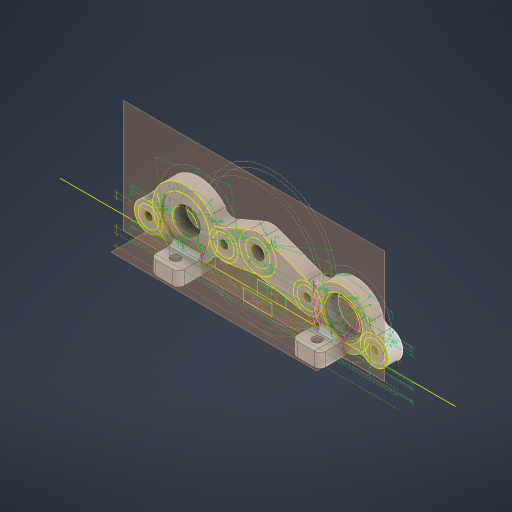
# Autodesk Inventor part: Motormount
Saved by Autodesk Inventor 2023.5 (Build 275446000, 446)
## iProperties
Created: 2024-12-07
Part Number: Motormount
Material: 一般
Document SubType Name: Modeling
Designer: IshiiLabHonda
Density: 1 g/cm^3
Appearance: 既定
Author: IshiiLabHonda
Autodesk Inventor part; units mm, degrees
ref_plane "YZ Plane" through (0, 0, 0) normal (1, 0, 0) x (0, 1, 0)
ref_plane "XZ Plane" through (0, 0, 0) normal (0, 1, 0) x (-1, 0, 0)
ref_plane "XY Plane" through (0, 0, 0) normal (0, 0, 1) x (1, 0, 0)
sketch "blueprint" plane through (0, 0, 0) normal (0, 0, 1) x (1, 0, 0)
  line L0 (0, 0) -> (0, 1) construction
  line L1 (0, 0) -> (1, 0) construction
  circle A0 centre (0, 0) radius 1.25
  circle A1 centre (0, 0) radius 11.5 construction
  line L2 (-25, -11.5) -> (25, -11.5) construction
  line L3 (-25, -9.5) -> (25, -9.5) construction
  line L4 (-25, -8.5) -> (25, -8.5) construction
  line L5 (-25, -4) -> (25, -4) construction
  circle A2 centre (0, 0) radius 10.65 construction
  circle A3 centre (-12.8817, -1.75) radius 2.25
  circle A4 centre (14.8916, -2.5) radius 4.35 construction
  circle A5 centre (14.8916, -2.5) radius 3.5 construction
  line L6 (-25, -3.2) -> (25, -3.2) construction
  circle A6 centre (-12.8817, -1.75) radius 4.25 construction
  circle A7 centre (-19.3421, -4.1014) radius 0.625 construction
  circle A8 centre (-6.0067, -1.75) radius 0.625 construction
  circle A9 centre (-12.8817, -1.75) radius 6.875 construction
  circle A10 centre (-19.3421, -4.1014) radius 1.825
  circle A11 centre (-6.0067, -1.75) radius 1.825
  circle A12 centre (14.8916, -2.5) radius 5
  circle A13 centre (14.8916, -2.5) radius 6.125 construction
  circle A14 centre (20.6472, -4.5949) radius 0.625 construction
  circle A15 centre (8.7666, -2.5) radius 0.625 construction
  circle A16 centre (20.6472, -4.5949) radius 1.825
  circle A17 centre (-19.3421, -4.1014) radius 0.8
  circle A18 centre (-6.0067, -1.75) radius 0.8
  circle A19 centre (20.6472, -4.5949) radius 0.8
  circle A20 centre (-19.3421, -4.1014) radius 2.5
  circle A21 centre (-6.0067, -1.75) radius 2.5
  circle A22 centre (20.6472, -4.5949) radius 2.5
  circle A23 centre (14.8916, -2.5) radius 3.6
  circle A24 centre (0, 0) radius 3.25
  line L7 (-15, -4) -> (-15, -8.5) construction
  line L8 (15, -4) -> (15, -8.5) construction
  line L9 (-10, -8.5) -> (-10, -6)
  line L10 (-15, -8.5) -> (-15, -6)
  line L11 (-15, -6) -> (-10, -6)
  line L12 (-12.5, -6) -> (-12.5, -8.5)
  line L13 (-13.3, -6) -> (-13.3, -8.5)
  line L14 (-11.7, -6) -> (-11.7, -8.5)
  line L15 (10, -8.5) -> (10, -6)
  line L16 (15, -8.5) -> (15, -6)
  line L17 (15, -6) -> (10, -6)
  line L18 (12.5, -6) -> (12.5, -8.5)
  line L19 (13.3, -6) -> (13.3, -8.5)
  line L20 (11.7, -6) -> (11.7, -8.5)
  line L21 (-15, -8.5) -> (-10, -8.5)
  line L22 (10, -8.5) -> (15, -8.5)
  circle A25 centre (8.7666, -2.5) radius 1.825
  line L23 (-12.8817, -1.75) -> (-19.3421, -4.1014) construction
  line L24 (-12.8817, -1.75) -> (-6.0067, -1.75) construction
  line L25 (14.8916, -2.5) -> (8.7666, -2.5) construction
  circle A26 centre (-12.8817, -1.75) radius 5.75
  line L26 (-2.5, -6.5) -> (2.5, -6.5)
  line L27 (2.5, -6.5) -> (2.5, -8.5)
  line L28 (2.5, -8.5) -> (-2.5, -8.5)
  line L29 (-2.5, -8.5) -> (-2.5, -6.5)
  line L30 (-2.5, -6.5) -> (2.5, -8.5) construction
  line L31 (2.5, -6.5) -> (-2.5, -8.5) construction
  line L32 (0, -6.5) -> (0, -8.5) construction
  line L33 (-0.8, -6.5) -> (-0.8, -8.5) construction
  line L34 (0.8, -6.5) -> (0.8, -8.5) construction
  circle A27 centre (8.7666, -2.5) radius 0.8
  circle A28 centre (8.7666, -2.5) radius 2.5
  line L35 (20.6472, -4.5949) -> (14.8916, -2.5) construction
  circle A29 centre (0, 0) radius 2.15
  circle A30 centre (14.8916, -2.5) radius 3 construction
  circle A31 centre (14.8916, -2.5) radius 3.2
  circle A32 centre (-12.8817, -1.75) radius 4.35
  point P0 (18.532, -5.9275)
  point P1 (19.8834, -2.2144)
  point P2 (0, -8.5)
  point P3 (-6.4807, -9.5)
  point P4 (6.4807, -9.5)
  point P5 (0, -7.5)
  point P6 (-17.257, -5.4808)
  point P7 (-7.4942, -3.7593)
  point P8 (-7.4942, 0.2593)
  point P9 (-18.6315, -1.7045)
  point P10 (11.284, 2.5721)
  point P11 (11.284, 2.0279)
  point P12 (16.9793, 5.3162)
  point P13 (16.5081, 5.5882)
  dimension "d0" = 1
  dimension "d1" = 1
  dimension "d2" = 2.5
  dimension "d3" = 23
  dimension "d4" = 50
  dimension "d5" = 50
  dimension "d6" = 2
  dimension "d7" = 50
  dimension "d9" = 1
  dimension "d10" = 50
  dimension "d12" = 4.5
  dimension "d13" = 21.3
  dimension "d14" = 4.5
  dimension "d15" = 8.7
  dimension "d17" = 0.1
  dimension "d18" = 0.1
  dimension "d20" = 7
  dimension "d21" = 50
  dimension "d22" = 0.8
  dimension "d23" = 8.5
  dimension "d26" = 1.25
  dimension "d27" = 1.25
  dimension "d28" = 1.2
  dimension "d29" = 1.2
  dimension "d31" = 1.5
  dimension "d32" = 1.25
  dimension "d33" = 1.25
  dimension "d34" = 1.2
  dimension "d37" = 0.5
  dimension "d40" = 1.6
  dimension "d41" = 1.6
  dimension "d43" = 1.6
  dimension "d49" = 2
  dimension "d56" = 30
  dimension "d90" = 2.5
  dimension "d92" = 5
  dimension "d93" = 1.6
  dimension "d104" = 1.2
  dimension "d105" = 5
  dimension "d106" = 1.6
  dimension "d107" = 2.5
  dimension "d129" = 5
  dimension "d130" = 5
  dimension "d132" = 5
  dimension "d155" = 25
  dimension "d158" = 1.5
  dimension "d160" = 0.5
  dimension "d161" = 200
  dimension "d166" = 1.6
  dimension "d167" = 5
  dimension "d168" = 2
  dimension "d178" = 1.6
  dimension "d179" = 5
  dimension "d187" = -2.8
  dimension "d196" = 4.3
  dimension "d218" = 12.0639
  dimension "d219" = 13.5411
  dimension "d220" = 200
  dimension "d237" = 0.1
  dimension "d238" = 6
  dimension "d239" = 0.2
  dimension "d247" = 0.1
  dimension "d257" = 9.75
  dimension "d258" = 9
  constraints: 70 end point, 33 centre point, 28 coincident, 16 point on line, 10 parallel, 8 midpoint, 7 vertical, 6 point on circle, 5 symmetric about line, 4 perpendicular, 3 horizontal, 1 tangent, 18 other
  measures "d0" distance of L0.start L0.end
  measures "d1" distance of L0.start L1.end
  measures "d2" diameter of A0
  measures "d3" diameter of A1
  measures "d4" distance of L2.start L2.end
  measures "d5" distance of L3.start L3.end
  measures "d6" distance between parallel lines of L2 L3
  measures "d7" distance of point (-25, -8.5) point (25, -8.5)
  measures "d10" distance of L5.start L5.end
  measures "d13" diameter of A2
  measures "d14" diameter of A3
  measures "d15" diameter of A4
  measures "d20" diameter of A5
  measures "d21" distance of L6.start L6.end
  measures "d22" distance between parallel lines of L5 L6
  measures "d23" diameter of A6
  measures "d26" diameter of A8
  measures "d27" diameter of A7
  measures "d28" radial gap between concentric circles of A10 A7
  measures "d29" radial gap between concentric circles of A11 A8
  measures "d31" radial gap between concentric circles of A12 A5
  measures "d32" diameter of A14
  measures "d33" diameter of A15
  measures "d34" radial gap between concentric circles of A14 A16
  measures "d40" diameter of A17
  measures "d41" diameter of A18
  measures "d43" diameter of A19
  measures "d49" radial gap between concentric circles of A24 A0
  measures "d56" distance between parallel lines of L8 L7
  measures "d90" distance of L10.start L10.end
  measures "d92" distance between parallel lines of L9 L10
  measures "d93" distance between parallel lines of L14 L13
  measures "d104" radial gap between concentric circles of A25 A15
  measures "d105" distance between parallel lines of L16 L15
  measures "d106" distance between parallel lines of L19 L20
  measures "d107" distance of L15.start L15.end
  measures "d129" diameter of A20
  measures "d130" diameter of A21
  measures "d132" diameter of A22
  measures "d155" distance between parallel lines of L18 L12
  measures "d158" radial gap between concentric circles of A26 A6
  measures "d166" distance between parallel lines of L33 L34
  measures "d167" distance between parallel lines of L27 L29
  measures "d168" distance between parallel lines of L26 L28
  measures "d178" diameter of A27
  measures "d179" diameter of A28
  measures "d187" distance edge to line of A6 L6
  measures "d196" diameter of A29
  measures "d218" distance of A14.centre L25.end
  measures "d219" distance of A7.centre A18.centre
  measures "d237" radial gap between concentric circles of A5 A23
  measures "d238" diameter of A30
  measures "d239" radial gap between concentric circles of A30 A31
  measures "d247" radial gap between concentric circles of A6 A32
  measures "d257" distance from line of L2 A3.centre
  measures "d258" distance from line of L2 A4.centre
sketch "スケッチ5" plane through (0, 0, 0) normal (0, 0, 1) x (1, 0, 0)
  circle A0 centre (0, 0) radius 10.65 construction
  circle A1 centre (0, 0) radius 11.5 construction
  line L0 (-25, -3.2) -> (25, -3.2) construction
  line L1 (-25, -4) -> (25, -4) construction
  line L2 (-25, -8.5) -> (25, -8.5) construction
  line L3 (-25, -9.5) -> (25, -9.5) construction
  line L4 (-25, -11.5) -> (25, -11.5) construction
  line L5 (0, 0) -> (1, 0) construction
  circle A2 centre (0, 0) radius 1.25 projected
  line L6 (0, 0) -> (0, 1) construction
  circle A3 centre (-6.0067, -1.75) radius 0.625 construction
  circle A4 centre (-6.0067, -1.75) radius 0.8 projected
  circle A5 centre (-6.0067, -1.75) radius 1.825 construction
  circle A6 centre (-6.0067, -1.75) radius 2.5 projected
  line L7 (-12.8817, -1.75) -> (-6.0067, -1.75) construction
  circle A7 centre (-12.8817, -1.75) radius 2.25 projected
  circle A8 centre (-12.8817, -1.75) radius 4.25 construction
  circle A9 centre (-12.8817, -1.75) radius 5.75 projected
  circle A10 centre (-12.8817, -1.75) radius 6.875 construction
  line L8 (-12.8817, -1.75) -> (-19.3421, -4.1014) construction
  circle A11 centre (-19.3421, -4.1014) radius 2.5 projected
  circle A12 centre (14.8916, -2.5) radius 3.5 construction
  circle A13 centre (14.8916, -2.5) radius 4.35 construction
  circle A14 centre (-19.3421, -4.1014) radius 0.625 construction
  circle A15 centre (-19.3421, -4.1014) radius 0.8 projected
  circle A16 centre (-19.3421, -4.1014) radius 1.825 construction
  circle A17 centre (14.8916, -2.5) radius 5 projected
  circle A18 centre (14.8916, -2.5) radius 6.125 construction
  circle A19 centre (20.6472, -4.5949) radius 0.625 construction
  circle A20 centre (8.7666, -2.5) radius 0.625 construction
  circle A21 centre (20.6472, -4.5949) radius 1.825 construction
  line L9 (14.8916, -2.5) -> (8.7666, -2.5) construction
  circle A22 centre (8.7666, -2.5) radius 0.8 projected
  circle A23 centre (8.7666, -2.5) radius 1.825 construction
  circle A24 centre (8.7666, -2.5) radius 2.5 projected
  circle A25 centre (14.8916, -2.5) radius 3.6 projected
  line L10 (20.6472, -4.5949) -> (14.8916, -2.5) construction
  circle A26 centre (20.6472, -4.5949) radius 2.5 projected
  circle A27 centre (20.6472, -4.5949) radius 0.8 projected
  line L11 (-10, -8.5) -> (-10, -6) projected
  line L12 (-11.7, -6) -> (-11.7, -8.5) projected
  line L13 (-15, -6) -> (-10, -6) projected
  line L14 (-12.5, -6) -> (-12.5, -8.5) projected
  line L15 (-13.3, -6) -> (-13.3, -8.5) projected
  line L16 (-15, -8.5) -> (-10, -8.5) projected
  line L17 (-15, -4) -> (-15, -8.5) construction
  line L18 (-15, -8.5) -> (-15, -6) projected
  line L19 (15, -4) -> (15, -8.5) construction
  line L20 (15, -8.5) -> (15, -6) projected
  line L21 (13.3, -6) -> (13.3, -8.5) projected
  line L22 (15, -6) -> (10, -6) projected
  line L23 (12.5, -6) -> (12.5, -8.5) projected
  line L24 (11.7, -6) -> (11.7, -8.5) projected
  line L25 (10, -8.5) -> (15, -8.5) projected
  line L26 (10, -8.5) -> (10, -6) projected
  circle A28 centre (0, 0) radius 3.25 projected
  line L27 (-2.5, -8.5) -> (-2.5, -6.5) projected
  line L28 (-0.8, -6.5) -> (-0.8, -8.5) construction
  line L29 (0, -6.5) -> (0, -8.5) construction
  line L30 (0.8, -6.5) -> (0.8, -8.5) construction
  line L31 (-2.5, -6.5) -> (2.5, -6.5) projected
  line L32 (-2.5, -6.5) -> (2.5, -8.5) construction
  line L33 (2.5, -6.5) -> (-2.5, -8.5) construction
  line L34 (2.5, -8.5) -> (-2.5, -8.5) projected
  line L35 (2.5, -6.5) -> (2.5, -8.5) projected
  line L36 (-15, -6) -> (-17.9261, 0.4132)
  line L37 (-10, -6) -> (-7.3501, 0.6797)
  line L38 (10, -6) -> (9.8941, -2.6584)
  line L39 (15, -6) -> (19.0045, 0.0357)
  line L40 (-5.6002, -4.2167) -> (0.5285, -3.2067)
  line L41 (-6.9886, 0.5491) -> (-1.2766, 2.9888)
  line L42 (1.1454, 3.0415) -> (9.6477, -0.1604)
  line L43 (-0.6311, -3.1881) -> (8.2811, -4.9524)
  point P0 (0, -7.5)
  point P1 (0, -8.5)
  point P2 (6.4807, -9.5)
  point P3 (-6.4807, -9.5)
  point P4 (10.2985, -4.4757)
  point P5 (9.9587, -4.6975)
  point P6 (0.8824, 3.1335)
  point P7 (-18.6315, -1.7045)
  point P8 (-17.257, -5.4808)
  point P9 (-7.4942, -3.7593)
  point P10 (18.532, -5.9275)
  point P11 (19.8834, -2.2144)
  point P12 (10.2985, -0.5243)
  point P13 (-7.4942, 0.2593)
  point P14 (18.0158, -1.9266)
  point P15 (-17.2201, -1.1342)
  point P16 (15, -7.4988)
  point P17 (11.3209, -6)
  point P18 (-0.053, -3.3026)
  point P19 (-15, -7.0956)
  point P20 (-10, -6.7258)
  point P21 (-7.5052, 0.2887)
  constraints: 16 end point, 8 point on circle, 8 tangent, 15 other
extrude "押し出し33" add sketch "スケッチ5" along normal blind 2.5 contours A6 A9 | A6 L41 A28 L43 L40 | A9 A6 L37 | A6 L37 A9 | A28 | A9 L11 L37 A6 | L40 A28 L42 A24 L43 | L37 A6 | A6 L37 L13 L18 A9 A11 | A9 L12 L13 L11 | A24 A17 L38 | A11 A9 | A9 A11 | A9 L14 L13 L12 | L38 A17 A24 | A24 A17 | A17 A26 L20 A25 L22 A24 | A9 L15 L13 L14 | L18 L13 L15 A9 | A26 A17 | A17 A26 | L22 L24 A17 | L24 L22 L23 A17 | A17 L21 L22 A25 L20 | L23 L22 L21 A17 | L20 L39 A25 | A25 L22 L20 | A25 L39 L22 | A7 | A15 | A27
extrude "押し出し34" cut sketch "blueprint" along normal blind 0.5 contours A10 A26 | A26 A10 | A26 A11 | A11 A26 | A16 A12 | A12 A16 | A25 A12 | A12 A25 | A17 | A19 | A29
extrude "押し出し39" add sketch "blueprint" along normal blind 6.5 contours A26 L13 L21 L10 | L10 L11 A32 L13 A26 | A26 L12 L21 L13 | L13 A32 L12 A26 | A26 L14 L11 L9 | L9 L21 L14 A26 | L11 L13 A32 | L13 L11 L12 A32 | A26 L14 L21 L12 | L12 A32 L11 L14 A26 | L12 L11 A32 | L16 L22 L19 A12 | A12 L19 L17 A23 L16 | L17 L20 A12 | A12 L20 L22 L15 L17 | L19 L22 L18 A12 | A12 L18 L17 L19 | A23 L17 L16 | L20 L17 L18 A12 | A12 L18 L22 L20 picked at (14.4705, -6.0203)
ref_plane "作業平面8" through (-15, -6, 2.5) normal (0, 1, 0) x (1, 0, 0)
sketch "スケッチ9" plane through (-15, -6, 2.5) normal (0, 1, 0) x (1, 0, 0)
  line L0 (0, 0) -> (5, 0) projected
  line L1 (0, 0) -> (0, -4) projected
  line L2 (5, -4) -> (0, -4) projected
  line L3 (5, 0) -> (5, -4) projected
  line L4 (26.3209, 0) -> (30, 0) projected
  line L5 (25, 2.5) -> (25, -4) projected
  line L6 (30, -4) -> (25, -4) projected
  line L7 (30, 0) -> (30, -4) projected
  line L8 (0, 2.5) -> (0, 0) projected
  line L9 (5, 2.5) -> (5, -4) projected
  line L10 (0, 0) -> (5, -4) construction
  line L11 (0, 2.5) -> (0, -4) projected
  line L12 (5, 0) -> (5.3524, 0) projected
  line L13 (0, -4) -> (5, 0) construction
  line L14 (30, 2.5) -> (30, -4) projected
  line L15 (25, 0) -> (30, -4) construction
  line L16 (25, 2.5) -> (25, -4) projected
  line L17 (30, 0) -> (30, 2.5) projected
  line L18 (25, -4) -> (30, 0) construction
  circle A0 centre (2.5, -2) radius 0.8
  circle A1 centre (27.5, -2) radius 0.8
  line L19 (26.3209, 2.5) -> (26.3209, 0) projected
  line L20 (26.3209, 2.5) -> (25, 2.5) projected
  point P0 (15, 2.5)
  dimension "d227" = 1.6
  dimension "d228" = 1.6
  constraints: 8 end point, 2 centre point, 2 midpoint
  measures "d227" diameter of A0
  measures "d228" diameter of A1
extrude "押し出し40" cut sketch "スケッチ9" against normal blind 6.5 contours A0 | A1
fillet "フィレット8" radius 1 4 edges at (-15, -7.25, 6.5) (-10, -7.25, 6.5) (10, -7.25, 6.5) (15, -7.25, 6.5)
fillet "フィレット9" radius 0.8 2 edges at (-12.5, -6, 2.5) (13.1604, -6, 2.5)
extrude "押し出し41" cut sketch "スケッチ5" along normal blind 6.5 contours A27
extrude "押し出し42" cut sketch "blueprint" along normal blind 6.5 contours L16 L17 A23 | A23 L17 L16 | A31
extrude "押し出し43" add sketch "blueprint" along normal up to surface (2.5 mm away) contours L16 L17 A23 | A23 L17 L16
ref_plane "作業平面9" through (0, 0, 2.5) normal (0, 0, 1) x (1, 0, 0)
sketch "スケッチ10" plane through (0, 0, 2.5) normal (0, 0, 1) x (1, 0, 0)
  line L0 (-1.2766, 2.9888) -> (-6.9886, 0.5491) projected
  arc A0 (-6.9886, 0.5491) -> (-7.4942, 0.2593) centre (-6.0067, -1.75) ccw projected
  line L1 (-1.2766, 2.9888) -> (-6.9886, 0.5491) projected
  line L2 (-5.6002, -4.2167) -> (0.5285, -3.2067) projected
  line L3 (-5.6002, -4.2167) -> (0.5285, -3.2067) projected
  circle A1 centre (-6.0067, -1.75) radius 0.8 projected
  circle A2 centre (-6.0067, -1.75) radius 0.8 projected
  circle A3 centre (-6.0067, -1.75) radius 1.825 projected
  circle A4 centre (-6.0067, -1.75) radius 1.825 projected
  arc A5 (-6.9886, 0.5491) -> (-7.4942, 0.2593) centre (-6.0067, -1.75) ccw projected
  arc A6 (-7.4942, -3.7593) -> (-5.6002, -4.2167) centre (-6.0067, -1.75) ccw projected
  arc A7 (-17.257, -5.4808) -> (-15, -7.0956) centre (-12.8817, -1.75) ccw projected
  arc A8 (-7.4942, -3.7593) -> (-5.6002, -4.2167) centre (-6.0067, -1.75) ccw projected
  arc A9 (-17.257, -5.4808) -> (-15, -7.0956) centre (-12.8817, -1.75) ccw projected
  arc A10 (0.5285, -3.2067) -> (-0.6311, -3.1881) centre (0, 0) ccw projected
  circle A11 centre (0, 0) radius 1.25 projected
  circle A12 centre (0, 0) radius 1.25 projected
  circle A13 centre (0, 0) radius 2.15 projected
  circle A14 centre (0, 0) radius 2.15 projected
  arc A15 (0.5285, -3.2067) -> (-0.6311, -3.1881) centre (0, 0) ccw projected
  arc A16 (0.5285, -3.2067) -> (-0.6311, -3.1881) centre (0, 0) ccw projected
  arc A17 (0.5285, -3.2067) -> (-0.6311, -3.1881) centre (0, 0) ccw projected
  line L4 (-0.6311, -3.1881) -> (8.2811, -4.9524) projected
  line L5 (9.6477, -0.1604) -> (1.1454, 3.0415) projected
  line L6 (9.6477, -0.1604) -> (1.1454, 3.0415) projected
  circle A18 centre (8.7666, -2.5) radius 0.8 projected
  circle A19 centre (8.7666, -2.5) radius 0.8 projected
  line L7 (-0.6311, -3.1881) -> (8.2811, -4.9524) projected
  line L8 (-15, -8.5) -> (-10, -8.5) projected
  line L9 (-10, -8.5) -> (-10, -6.9556) projected
  line L10 (-10, -6) -> (-10, -5.2) projected
  arc A20 (-15, -7.0868) -> (-15.4511, -5.0113) centre (-20, -7.0868) ccw projected
  arc A21 (-15, -7.0868) -> (-15.4511, -5.0113) centre (-20, -7.0868) ccw projected
  line L11 (-15, -7.0956) -> (-15, -5.2) projected
  line L12 (-10, -8.5) -> (-10, -6) projected
  line L13 (-15, -5.2) -> (-15, -6) projected
  line L14 (-15, -6) -> (-10, -6) projected
  line L15 (-11, -6) -> (-11, -8.5) projected
  line L16 (-10, -8.5) -> (-11, -8.5) projected
  line L17 (-11, -6) -> (-14, -6) projected
  line L18 (-14, -8.5) -> (-11, -8.5) projected
  line L19 (-15, -6) -> (-15, -8.5) projected
  line L20 (-14, -8.5) -> (-14, -6) projected
  line L21 (-15, -6) -> (-14, -6) projected
  line L22 (-15, -7.0868) -> (-15, -8.5) projected
  arc A22 (10.2985, -0.5243) -> (9.6477, -0.1604) centre (8.7666, -2.5) ccw projected
  arc A23 (19.8834, -2.2144) -> (10.2985, -0.5243) centre (14.8916, -2.5) ccw projected
  arc A24 (18.532, -5.9275) -> (19.8834, -2.2144) centre (20.6472, -4.5949) ccw projected
  arc A25 (19.8834, -2.2144) -> (10.2985, -0.5243) centre (14.8916, -2.5) ccw projected
  arc A26 (10.2985, -0.5243) -> (9.6477, -0.1604) centre (8.7666, -2.5) ccw projected
  circle A27 centre (20.6472, -4.5949) radius 1.825 projected
  circle A28 centre (20.6472, -4.5949) radius 1.825 projected
  circle A29 centre (14.8916, -2.5) radius 3.2 projected
  circle A30 centre (14.8916, -2.5) radius 3.2 projected
  arc A31 (10.2985, -4.4757) -> (10.6833, -5.2) centre (14.8916, -2.5) ccw projected
  arc A32 (10.2985, -0.5243) -> (9.6477, -0.1604) centre (8.7666, -2.5) ccw projected
  arc A33 (19.8834, -2.2144) -> (10.2985, -0.5243) centre (14.8916, -2.5) ccw projected
  circle A34 centre (20.6472, -4.5949) radius 0.8 projected
  arc A35 (18.532, -5.9275) -> (19.8834, -2.2144) centre (20.6472, -4.5949) ccw projected
  circle A36 centre (20.6472, -4.5949) radius 0.8 projected
  line L23 (-10, -5.2) -> (-10, -6.7258) projected
  arc A37 (-9.6476, -5.1118) -> (-10, -6.9556) centre (-5, -6.9556) ccw projected
  arc A38 (-9.6476, -5.1118) -> (-10, -6.9556) centre (-5, -6.9556) ccw projected
  line L24 (-14, -8.5) -> (-15, -8.5) projected
  line L25 (-11.7, -8.5) -> (-13.3, -8.5) projected
  line L26 (-13.3, -6) -> (-11.7, -6) projected
  line L27 (9.8782, 0.5881) -> (10.0005, -6.0244) projected
  line L28 (10, -8.5) -> (15, -8.5) projected
  line L29 (15, -8.5) -> (15, -7.5078) projected
  line L30 (15.8336, -4.7436) -> (19.0045, 0.0357) projected
  arc A39 (15.8336, -4.7436) -> (15, -7.5078) centre (20, -7.5078) ccw projected
  line L31 (15.8336, -4.7436) -> (19.0045, 0.0357) projected
  arc A40 (8.2811, -4.9524) -> (10.2985, -4.4757) centre (8.7666, -2.5) ccw projected
  line L32 (15, -6) -> (15, -5.2) projected
  line L33 (9.8782, 0.5881) -> (9.9852, -5.2) projected
  arc A41 (15.8336, -4.7436) -> (15, -7.5078) centre (20, -7.5078) ccw projected
  line L34 (15, -5.2) -> (15, -7.5078) projected
  line L35 (12.5104, -5.2) -> (10.6833, -5.2) projected
  line L36 (11.7, -6) -> (13.3, -6) projected
  line L37 (11.3209, -6) -> (14.049, -6) projected
  line L38 (9.9852, -5.2) -> (10.0005, -6.0244) projected
  line L39 (15, -8.5) -> (15, -6) projected
  line L40 (13.3, -8.5) -> (11.7, -8.5) projected
  line L41 (10, -6) -> (10, -8.5) projected
  line L42 (10, -6) -> (10, -8.5) projected
  arc A42 (-7.4942, 0.2593) -> (-18.6315, -1.7045) centre (-12.8817, -1.75) ccw projected
  arc A43 (-18.6315, -1.7045) -> (-17.257, -5.4808) centre (-19.3421, -4.1014) ccw projected
  line L43 (-17.9261, 0.4132) -> (-15.4511, -5.0113) projected
  circle A44 centre (-19.3421, -4.1014) radius 1.825 projected
  circle A45 centre (-19.3421, -4.1014) radius 1.825 projected
  circle A46 centre (8.7666, -2.5) radius 1.825 projected
  circle A47 centre (8.7666, -2.5) radius 1.825 projected
  line L44 (-9.6476, -5.1118) -> (-7.3501, 0.6797) projected
  line L45 (-9.6476, -5.1118) -> (-7.3501, 0.6797) projected
  arc A48 (-7.4942, 0.2593) -> (-18.6315, -1.7045) centre (-12.8817, -1.75) ccw projected
  line L46 (-17.9261, 0.4132) -> (-15.4511, -5.0113) projected
  arc A49 (-18.6315, -1.7045) -> (-17.257, -5.4808) centre (-19.3421, -4.1014) ccw projected
  line L47 (-10, -5.2) -> (-15, -5.2) projected
  line L48 (-11, -6) -> (-10, -6) projected
  line L49 (11, -8.5) -> (10, -8.5) projected
  line L50 (11, -8.5) -> (14, -8.5) projected
  line L51 (11, -8.5) -> (11, -6) projected
  line L52 (15, -8.5) -> (14, -8.5) projected
  line L53 (14, -6) -> (14, -8.5) projected
  line L54 (14, -6) -> (15, -6) projected
  line L55 (14, -6) -> (11, -6) projected
  line L56 (11.3209, -6) -> (11, -6) projected
  line L57 (-35, -6) -> (35, -6) projected
  line L58 (-25, -3.2) -> (25, -3.2) construction
  line L59 (-25, -4) -> (25, -4) construction
  line L60 (-25, -8.5) -> (25, -8.5) construction
  line L61 (-25, -9.5) -> (25, -9.5) construction
  line L62 (-25, -11.5) -> (25, -11.5) construction
  circle A50 centre (0, 0) radius 10.65 construction
  circle A51 centre (0, 0) radius 11.5 construction
  circle A52 centre (0, 0) radius 1.25 projected
  circle A53 centre (0, 0) radius 3.25 projected
  line L63 (-2.5, -8.5) -> (-2.5, -6.5) projected
  line L64 (-0.8, -6.5) -> (-0.8, -8.5) construction
  circle A54 centre (0, 0) radius 2.15 projected
  line L65 (0, -6.5) -> (0, -8.5) construction
  line L66 (0.8, -6.5) -> (0.8, -8.5) construction
  line L67 (-2.5, -6.5) -> (2.5, -6.5) projected
  line L68 (2.5, -8.5) -> (-2.5, -8.5) projected
  line L69 (2.5, -6.5) -> (-2.5, -8.5) construction
  line L70 (-2.5, -6.5) -> (2.5, -8.5) construction
  circle A55 centre (-6.0067, -1.75) radius 0.625 construction
  circle A56 centre (-6.0067, -1.75) radius 0.8 projected
  circle A57 centre (-6.0067, -1.75) radius 1.825 projected
  circle A58 centre (-6.0067, -1.75) radius 2.5 projected
  line L71 (-15, -4) -> (-15, -8.5) construction
  line L72 (-15, -8.5) -> (-15, -6) projected
  line L73 (-13.3, -6) -> (-13.3, -8.5) projected
  line L74 (-12.5, -6) -> (-12.5, -8.5) projected
  line L75 (-15, -6) -> (-10, -6) projected
  line L76 (-11.7, -6) -> (-11.7, -8.5) projected
  line L77 (-15, -8.5) -> (-10, -8.5) projected
  line L78 (-10, -8.5) -> (-10, -6) projected
  circle A59 centre (-12.8817, -1.75) radius 2.25 projected
  circle A60 centre (-12.8817, -1.75) radius 4.25 construction
  line L79 (-12.8817, -1.75) -> (-6.0067, -1.75) construction
  circle A61 centre (-12.8817, -1.75) radius 5.75 projected
  line L80 (-12.8817, -1.75) -> (-19.3421, -4.1014) construction
  circle A62 centre (-19.3421, -4.1014) radius 0.625 construction
  circle A63 centre (-19.3421, -4.1014) radius 1.825 projected
  circle A64 centre (-19.3421, -4.1014) radius 2.5 projected
  circle A65 centre (-19.3421, -4.1014) radius 0.8 projected
  line L81 (2.5, -6.5) -> (2.5, -8.5) projected
  line L82 (15, -6) -> (10, -6) projected
  line L83 (10, -8.5) -> (10, -6) projected
  line L84 (10, -8.5) -> (15, -8.5) projected
  line L85 (15, -4) -> (15, -8.5) construction
  line L86 (15, -8.5) -> (15, -6) projected
  line L87 (11.7, -6) -> (11.7, -8.5) projected
  line L88 (12.5, -6) -> (12.5, -8.5) projected
  line L89 (13.3, -6) -> (13.3, -8.5) projected
  circle A66 centre (14.8916, -2.5) radius 5 projected
  circle A67 centre (14.8916, -2.5) radius 6.125 construction
  circle A68 centre (20.6472, -4.5949) radius 0.625 construction
  circle A69 centre (8.7666, -2.5) radius 0.625 construction
  circle A70 centre (20.6472, -4.5949) radius 1.825 projected
  circle A71 centre (20.6472, -4.5949) radius 0.8 projected
  circle A72 centre (20.6472, -4.5949) radius 2.5 projected
  line L90 (14.8916, -2.5) -> (8.7666, -2.5) construction
  circle A73 centre (8.7666, -2.5) radius 1.825 projected
  circle A74 centre (8.7666, -2.5) radius 2.5 projected
  circle A75 centre (14.8916, -2.5) radius 3 construction
  circle A76 centre (14.8916, -2.5) radius 3.2 projected
  circle A77 centre (14.8916, -2.5) radius 3.6 projected
  line L91 (20.6472, -4.5949) -> (14.8916, -2.5) construction
  circle A78 centre (8.7666, -2.5) radius 0.8 projected
  line L92 (0, 0) -> (0, 1) construction
  line L93 (0, 0) -> (1, 0) construction
  circle A79 centre (14.8916, -2.5) radius 3.5 construction
  circle A80 centre (14.8916, -2.5) radius 4.35 construction
  line L94 (12.5, -6) -> (12.5, -8.5) projected
  line L95 (11.7, -6) -> (11.7, -8.5) projected
  line L96 (13.3, -6) -> (13.3, -8.5) projected
  line L97 (10, -8.5) -> (10, -6) projected
  line L98 (10, -8.5) -> (15, -8.5) projected
  line L99 (15, -4) -> (15, -8.5) construction
  line L100 (15, -6) -> (10, -6) projected
  line L101 (15, -6) -> (19.0045, 0.0357) projected
  line L102 (10, -6) -> (9.8941, -2.6584) projected
  line L103 (14.8916, -2.5) -> (8.7666, -2.5) construction
  line L104 (-0.6311, -3.1881) -> (8.2811, -4.9524) projected
  line L105 (1.1454, 3.0415) -> (9.6477, -0.1604) projected
  circle A81 centre (0, 0) radius 10.65 construction
  circle A82 centre (0, 0) radius 11.5 construction
  line L106 (-25, -11.5) -> (25, -11.5) construction
  line L107 (-25, -9.5) -> (25, -9.5) construction
  line L108 (-25, -8.5) -> (25, -8.5) construction
  line L109 (-25, -4) -> (25, -4) construction
  line L110 (-25, -3.2) -> (25, -3.2) construction
  circle A83 centre (8.7666, -2.5) radius 0.625 construction
  circle A84 centre (8.7666, -2.5) radius 0.8 projected
  circle A85 centre (8.7666, -2.5) radius 1.825 construction
  circle A86 centre (8.7666, -2.5) radius 2.5 projected
  line L111 (-15, -6) -> (-17.9261, 0.4132) projected
  line L112 (-10, -6) -> (-7.3501, 0.6797) projected
  line L113 (-12.8817, -1.75) -> (-6.0067, -1.75) construction
  circle A87 centre (-19.3421, -4.1014) radius 0.625 construction
  circle A88 centre (-19.3421, -4.1014) radius 0.8 projected
  circle A89 centre (-19.3421, -4.1014) radius 1.825 construction
  circle A90 centre (-19.3421, -4.1014) radius 2.5 projected
  line L114 (-12.8817, -1.75) -> (-19.3421, -4.1014) construction
  circle A91 centre (-12.8817, -1.75) radius 5.75 projected
  circle A92 centre (-12.8817, -1.75) radius 4.25 construction
  circle A93 centre (-12.8817, -1.75) radius 2.25 projected
  circle A94 centre (14.8916, -2.5) radius 3.5 construction
  circle A95 centre (14.8916, -2.5) radius 4.35 construction
  circle A96 centre (14.8916, -2.5) radius 5 projected
  circle A97 centre (14.8916, -2.5) radius 6.125 construction
  circle A98 centre (20.6472, -4.5949) radius 0.625 construction
  circle A99 centre (20.6472, -4.5949) radius 1.825 construction
  circle A100 centre (14.8916, -2.5) radius 3.6 projected
  line L115 (20.6472, -4.5949) -> (14.8916, -2.5) construction
  circle A101 centre (20.6472, -4.5949) radius 0.8 projected
  circle A102 centre (20.6472, -4.5949) radius 2.5 projected
  line L116 (-15, -6) -> (-10, -6) projected
  line L117 (-15, -4) -> (-15, -8.5) construction
  line L118 (-15, -8.5) -> (-10, -8.5) projected
  line L119 (-15, -8.5) -> (-15, -6) projected
  line L120 (-13.3, -6) -> (-13.3, -8.5) projected
  line L121 (-12.5, -6) -> (-12.5, -8.5) projected
  line L122 (-11.7, -6) -> (-11.7, -8.5) projected
  line L123 (-10, -8.5) -> (-10, -6) projected
  line L124 (0, 0) -> (1, 0) construction
  circle A103 centre (0, 0) radius 1.25 projected
  line L125 (0, 0) -> (0, 1) construction
  circle A104 centre (-6.0067, -1.75) radius 0.625 construction
  circle A105 centre (-6.0067, -1.75) radius 0.8 projected
  circle A106 centre (-6.0067, -1.75) radius 1.825 construction
  circle A107 centre (-6.0067, -1.75) radius 2.5 projected
  line L126 (-5.6002, -4.2167) -> (0.5285, -3.2067) projected
  line L127 (-2.5, -8.5) -> (-2.5, -6.5) projected
  line L128 (-0.8, -6.5) -> (-0.8, -8.5) construction
  line L129 (0, -6.5) -> (0, -8.5) construction
  line L130 (0.8, -6.5) -> (0.8, -8.5) construction
  line L131 (-6.9886, 0.5491) -> (-1.2766, 2.9888) projected
  circle A108 centre (0, 0) radius 3.25 projected
  line L132 (2.5, -6.5) -> (2.5, -8.5) projected
  line L133 (-2.5, -6.5) -> (2.5, -8.5) construction
  line L134 (2.5, -6.5) -> (-2.5, -8.5) construction
  line L135 (2.5, -8.5) -> (-2.5, -8.5) projected
  line L136 (-2.5, -6.5) -> (2.5, -6.5) projected
  line L137 (15, -8.5) -> (15, -6) projected
  circle A109 centre (-12.8817, -1.75) radius 4.35 projected
  point P0 (0.8824, 3.1335)
  point P1 (-17.2201, -1.1342)
  point P2 (0, -8.5)
  point P3 (0, -7.5)
  point P4 (6.4807, -9.5)
  point P5 (-6.4807, -9.5)
  point P6 (-6.4807, -9.5)
  point P7 (6.4807, -9.5)
  point P8 (0, -8.5)
  point P9 (0, -7.5)
  constraints: 68 other
extrude "押し出し45" cut sketch "スケッチ10" against normal blind 0.5 contours A77 A39 L57 | L57 A39 A29 L30 A77 | A77 L30 A29 L32 L54 | L57 L101 A29 A39 | A39 A77 L34 L57 | A77 L54 L34 | L32 A29 L101
extrude "押し出し46" cut sketch "スケッチ10" against normal blind 0.5 contours A109 L44 | L44 A109 L47 L11 L111 L43 | A109 L14 L11 L47 | L43 A20 A109 | A109 L74 L14 | L111 A109 A20 | L74 A109 L73 L14 | L14 L73 A109 | A59
fillet "フィレット10" radius 2 6 edges at (-18.6315, -1.7045, 1.25) (-7.4942, 0.2593, 1.25) (-7.4942, -3.7593, 1.25) (10.2985, -0.5243, 1.25) (19.8834, -2.2144, 1.25) (18.532, -5.9275, 1.25)
extrude "押し出し47" add sketch "blueprint" along normal blind 0.5 contours A29
extrude "押し出し48" cut sketch "スケッチ5" along normal blind 10 contours A7
extrude "押し出し49" cut sketch "スケッチ5" along normal blind 10 contours A15
equation "\"d5\" = d4"
equation "\"d7\" = d4"
equation "\"d10\" = d4"
